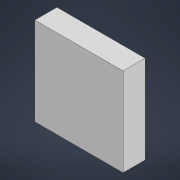
# Autodesk Inventor part: Clip_MarkerHolderV1
Saved by Autodesk Inventor 2022 (Build 260153000, 153)
## iProperties
Created: 2023-05-06
Part Number: Clip_MarkerHolderV1
Material: Generic
Document SubType Name: Modeling
Designer: Karl Spiteri
Density: 1 g/cm^3
Appearance: Default
Author: Karl Spiteri
Autodesk Inventor part; units mm, degrees
ref_plane "YZ Plane" through (0, 0, 0) normal (1, 0, 0) x (0, 1, 0)
ref_plane "XZ Plane" through (0, 0, 0) normal (0, 1, 0) x (-1, 0, 0)
ref_plane "XY Plane" through (0, 0, 0) normal (0, 0, 1) x (1, 0, 0)
sketch "Sketch5" plane through (0, 0, 0) normal (0, 0, 1) x (1, 0, 0)
  circle A0 centre (0, 0) radius 14.35
  circle A1 centre (0, 0) radius 17.15
  line L0 (0, 0) -> (20, 0)
  line L1 (20, 0) -> (20, 20)
  line L2 (20, 20) -> (0, 20)
  line L3 (0, 20) -> (0, 0)
  line L4 (20, 20) -> (-20, 20)
  line L5 (-20, 20) -> (-20, -20)
  line L6 (-20, -20) -> (20, -20)
  line L7 (20, -20) -> (20, 20)
  dimension "d36" = 28.7
  dimension "d37" = 34.3
  dimension "d54" = 20
  dimension "d55" = 20
  dimension "d56" = 40
  dimension "d57" = 40
  constraints: 16 end point, 4 parallel, 2 centre point, 2 coincident, 2 horizontal, 2 perpendicular
  measures "d36" diameter of A0
  measures "d37" diameter of A1
  measures "d54" distance of L2.end L1.end
  measures "d55" distance of L1.end L0.end
  measures "d56" distance of L6.end L5.end
  measures "d57" distance of L5.end L4.end
extrude "Extrusion10" add sketch "Sketch5" along normal blind 10
sketch "Sketch8" plane through (0, 0, 0) normal (0, 0, -1) x (-1, 0, 0)
  circle A0 centre (0, 0) radius 14.35
  circle A1 centre (0, 0) radius 17.15
  circle A2 centre (0, 0) radius 14.35
  circle A3 centre (0, 0) radius 17.15
  dimension "d60" = 28.7
  dimension "d61" = 34.3
  dimension "d62" = 28.7
  dimension "d63" = 34.3
  constraints: 4 centre point, 4 coincident
  measures "d60" diameter of A0
  measures "d61" diameter of A1
  measures "d62" diameter of A2
  measures "d63" diameter of A3
extrude "Extrusion11" cut sketch "Sketch8" against normal blind 5
body "Solid3"
